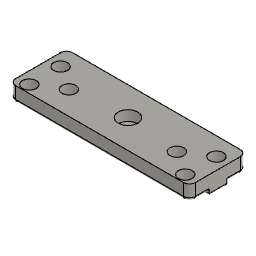
10X15 Y Cable Chain Mount MOD v3 (Autodesk Fusion 360 design; units mm, degrees)
Autodesk Fusion 360 part; units mm, degrees
sketch "草图1" plane through (0, 0, 0) normal (0, 0, 1) x (1, 0, 0)
  line L0 (0, 0) -> (60, 0)
  line L1 (60, 0) -> (60, 19)
  line L2 (60, 19) -> (0, 19)
  line L3 (0, 19) -> (0, 0)
  line L4 (0, 9.5) -> (60, 9.5) construction
  line L5 (0, 12.44) -> (60, 12.44)
  line L6 (60, 12.44) -> (60, 6.56)
  line L7 (60, 6.56) -> (0, 6.56)
  line L8 (0, 6.56) -> (0, 12.44)
  line L9 (0, 12.44) -> (60, 6.56) construction
  line L10 (60, 12.44) -> (0, 6.56) construction
  point P0 (30, 9.5)
  point P1 (30, 9.5)
  dimension "d1" = 60
  dimension "d2" = 19
  dimension "d3" = 60
  dimension "d4" = 5.88
  constraint horizontal L0
  constraint vertical L1
  constraint horizontal L2
  constraint vertical L3
  constraint coincident L0.start L3.end
  constraint midpoint L3 L4.start
  constraint midpoint L1 L4.end
  constraint horizontal L5
  constraint perpendicular L5 L6
  constraint parallel L5 L7
  constraint parallel L6 L8
  constraint coincident L9 P1
  constraint coincident L10 P1
  constraint midpoint L4 P1
  constraint coincident P1 P0
  measures "d1" distance of L0.start L0.end
  measures "d2" distance of L0.start L2.end
  measures "d3" distance of L6.end L7.end
  measures "d4" distance of L5.end L6.end
extrude "拉伸1" add sketch "草图1" along normal blind 5
extrude "拉伸2" add sketch "草图1" against normal blind 1 contours L1 L3 L5 L6 L7 L8
sketch "草图2" plane through (0, 0, 5) normal (0, 0, 1) x (-1, 0, 0)
  line L0 (0, 0) -> (-60, 0)
  line L1 (-60, 0) -> (-60, -19)
  line L2 (-60, -19) -> (0, -19)
  line L3 (0, -19) -> (0, 0)
  point P0 (-30, -9.5)
hole "孔1" at (30, 9.5, 5) direction (0, 0, -1) diameter 3.2 depth 8 tip angle 180 counterbore diameter 6.5 counterbore depth 3.4
sketch "草图4" plane through (0, 0, 5) normal (0, 0, 1) x (-1, 0, 0)
  circle A0 centre (-30, -9.5) radius 3.25
  line L0 (0, 0) -> (-60, 0)
  line L1 (-60, 0) -> (-60, -19)
  line L2 (-60, -19) -> (0, -19)
  line L3 (0, -19) -> (0, 0)
  line L4 (-40.689, -19) -> (-40.689, 3.3911)
  circle A1 centre (-56, -2.6) radius 2.3
  circle A2 centre (-56, -13) radius 2.3
  circle A3 centre (-48, -7.8) radius 2.3
  line L5 (-40.689, 3.3911) -> (-60, 3.3911)
  line L6 (-60, -19) -> (-40.689, -19)
  line L7 (-60, 3.3911) -> (-60, -19)
  line L8 (-19.311, -19) -> (0, -19)
  line L9 (-19.311, 3.3911) -> (-19.311, -19)
  line L10 (0, -19) -> (0, 3.3911)
  line L11 (0, 3.3911) -> (-19.311, 3.3911)
  circle A4 centre (-4, -2.6089) radius 2.3
  circle A5 centre (-12, -7.8089) radius 2.3
  circle A6 centre (-4, -13.0089) radius 2.3
  point P0 (-60, -19)
  point P1 (-60, -19)
  dimension "d14" = 4.6
  dimension "d15" = 4.6
  dimension "d16" = 4.6
  dimension "d17" = 4.6
  dimension "d18" = 4.6
  dimension "d19" = 4.6
  constraint horizontal L6
  constraint vertical L4
  constraint horizontal L5
  constraint vertical L7
  constraint coincident P1 P0
  measures "d14" diameter of A5
  measures "d15" diameter of A4
  measures "d16" diameter of A6
  measures "d17" diameter of A3
  measures "d18" diameter of A2
  measures "d19" diameter of A1
extrude "拉伸3" cut sketch "草图4" against normal blind 3.8 contours A1 | A2 | A3 | A4 | A5 | A6
fillet "圆角1" radius 2 4 edges at (60, 0, 2.5) (60, 19, 2.5) (0, 19, 2.5) (0, 0, 2.5)
fillet "圆角2" radius 0.5 4 edges at (60, 9.5, -1) (30, 6.56, -1) (30, 12.44, -1) (0, 9.5, -1)
fillet "圆角3" radius 1 10 edges at (0, 4.28, 0) (0.5858, 0.5858, 0) (30, 0, 0) (59.4142, 0.5858, 0) (60, 4.28, 0) (60, 14.72, 0) (59.4142, 18.4142, 0) (30, 19, 0) (0.5858, 18.4142, 0) (0, 14.72, 0)
